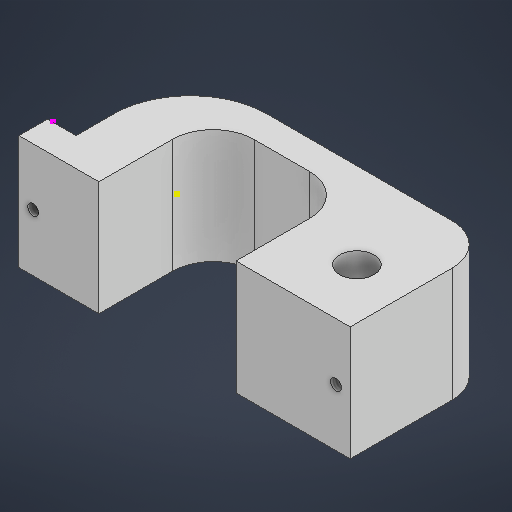
# Autodesk Inventor part: chassis3
Saved by Autodesk Inventor 2027 (Build 310192060, 192F)
## iProperties
Created: 2026-07-01
Part Number: chassis3
Material: Generic
Document SubType Name: Modeling
Designer: loren
Density: 1 g/cm^3
Appearance: Default
Author: loren
Autodesk Inventor part; units mm, degrees
ref_plane "YZ Plane" through (0, 0, 0) normal (1, 0, 0) x (0, 1, 0)
ref_plane "XZ Plane" through (0, 0, 0) normal (0, 1, 0) x (-1, 0, 0)
ref_plane "XY Plane" through (0, 0, 0) normal (0, 0, 1) x (1, 0, 0)
sketch "Sketch1" plane through (0, 0, 0) normal (0, 1, 0) x (-1, 0, 0)
  line L0 (4.35, -5) -> (-7.65, -5)
  line L1 (-7.65, -5) -> (-7.65, 5)
  line L2 (-7.65, 5) -> (4.35, 5)
  line L3 (4.35, 5) -> (4.35, -5)
  line L4 (4.35, -5) -> (-7.65, 5) construction
  line L5 (-7.65, -5) -> (4.35, 5) construction
  line L6 (4.35, 5) -> (11.35, 5)
  line L7 (11.35, 5) -> (11.35, 2.5)
  line L8 (11.35, 2.5) -> (8.85, 2.5)
  line L9 (8.85, 2.5) -> (8.85, -7.5)
  line L10 (-7.45, 2.5) -> (-7.45, -7.5)
  line L11 (-7.45, -7.5) -> (8.85, -7.5)
  line L12 (-7.65, 5) -> (-7.45, 5)
  line L13 (-7.45, 5) -> (-7.45, 2.5)
  line L14 (-17.65, 5) -> (-17.65, -7.5)
  line L15 (-17.65, -7.5) -> (-7.45, -7.5)
  line L16 (-17.65, 5) -> (-7.45, 5)
  circle A0 centre (-13.23, 0) radius 1.5
  point P0 (-7.45, -5)
  dimension "d29" = 10
  dimension "d30" = 7
  dimension "d31" = 2.5
  dimension "d32" = 2.5
  dimension "d33" = 10
  dimension "d34" = 90
  dimension "d35" = 10
  dimension "d40" = 12
  dimension "d46" = 3
  dimension "d52" = 24.58
  constraints: 34 end point, 6 perpendicular, 3 horizontal, 2 collinear, 2 parallel, 2 vertical, 1 centre point, 1 point on line
  measures "d29" distance of L0.end L1.end
  measures "d30" distance of L2.end L6.end
  measures "d31" distance of L6.end L7.end
  measures "d32" distance of L7.end L8.end
  measures "d33" distance of L8.end L9.end
  measures "d34" angle of L9 L8
  measures "d35" distance of L10.start L10.end
  measures "d40" distance of L1.end L2.end
  measures "d46" diameter of A0
  measures "d52" horizontal distance of A0.centre L6.end
extrude "Extrusion9" add sketch "Sketch1" against normal blind 10 contours L3 L6 L7 L8 L9 L11 L10 L0 | L10 L15 L14 L16 L1 L0
fillet "Fillet7" radius 3.5875 2 edges at (-4.35, -5, -5) (7.65, -5, -5)
fillet "Fillet9" radius 3.5875 1 edges at (17.65, -5, -7.5)
fillet "Fillet10" radius 6.7625 1 edges at (-8.85, -5, -7.5)
sketch "Sketch5" plane through (-11.35, -10, 2.5) normal (0, 0, -1) x (-1, 0, 0)
  line L0 (-0.5, 0) -> (-0.5, 10) projected
  point P0 (-11.35, 10)
  point P1 (-0.5, 5)
  constraints: 1 midpoint
sketch "Sketch6" plane through (-8.85, 0, 2.5) normal (0, 0, -1) x (-1, 0, 0)
  line L0 (2.5, -10) -> (0, -10) projected
  point P0 (-8.85, 0)
  point P1 (1.25, -5)
hole "Hole1" at (-10.1, -5, 2.5) direction (0, 0, 1) diameter 0.9398 depth 3.65 tip angle 118 thread size "120-102 UNM" class "2B" standard "ANSI Unified Screw Threads"
sketch "Sketch7" plane through (7.65, 0, 5) normal (0, 0, 1) x (1, 0, 0)
  point P0 (-7.65, 0)
  point P1 (8.75, -5)
hole "Hole2" at (16.4, -5, 5) direction (0, 0, -1) diameter 0.9398 depth 3.65 tip angle 118 thread size "120-102 UNM" class "2B" standard "ANSI Unified Screw Threads"
body "Solid5"
